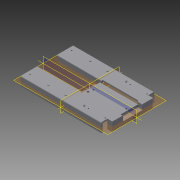
# Autodesk Inventor part: KarosserieDachTeil1
Saved by Autodesk Inventor 2015 (Build 190159000, 159)
## iProperties
Created: 2018-12-10
Part Number: KarosserieDachTeil1
Material: Generisch
Document SubType Name: Modeling
Designer: Boris
Density: 1 g/cm^3
Appearance: Vorgabe
Author: Boris
Autodesk Inventor part; units mm, degrees
sketch "Skizze1" plane through (0, 0, 0) normal (0, 0, 1) x (1, 0, 0)
  line L0 (-123.688, 77) -> (123.688, 77)
  line L1 (123.688, 77) -> (123.688, -77)
  line L2 (123.688, -77) -> (-123.688, -77)
  line L3 (-123.688, -77) -> (-123.688, 77)
  line L4 (-173.1632, 0) -> (173.1632, 0) projected
  line L5 (0, 107.8) -> (0, -107.8) projected
  point P0 (0, 0)
  dimension "d0" = 247.376
  dimension "d1" = 154
  constraints: 8 end point, 2 parallel, 1 horizontal, 1 perpendicular, 2 other
  measures "d0" distance of L1.end L2.end
  measures "d1" distance of L0.end L1.end
extrude "Extrusion1" add sketch "Skizze1" along normal mid plane 27
sketch "Skizze2" plane through (0, 0, -13.5) normal (0, 0, -1) x (-1, 0, 0)
  line L0 (123.688, -73) -> (-123.688, -73)
  line L1 (173.1632, 0) -> (-173.1632, 0) projected
  line L2 (123.688, -31) -> (-123.688, -31)
  line L3 (-123.688, -77) -> (123.688, -77) projected
  line L4 (123.688, 73) -> (-123.688, 73)
  line L5 (123.688, 31) -> (-123.688, 31)
  line L6 (123.688, -73) -> (123.688, -31)
  line L7 (0, -107.8) -> (0, 107.8) projected
  line L8 (-123.688, -73) -> (-123.688, -31)
  line L9 (123.688, 73) -> (123.688, 31)
  line L10 (-123.688, 73) -> (-123.688, 31)
  point P0 (0, 0)
  dimension "d4" = 4
  dimension "d5" = 42
  dimension "d8" = 123.688
  dimension "d13" = 123.688
  constraints: 16 end point, 4 symmetric about line, 1 horizontal, 1 parallel, 1 vertical
  measures "d4" distance between parallel lines of L3 L0
  measures "d5" distance between parallel lines of L0 L2
  measures "d8" distance between parallel lines of L7 L6
  measures "d13" distance between parallel lines of L8 L7
extrude "Extrusion2" cut sketch "Skizze2" against normal blind 23
sketch "Skizze3" plane through (0, 0, 13.5) normal (0, 0, 1) x (1, 0, 0)
  line L0 (-123.688, 31) -> (123.688, 31) projected
  line L1 (123.688, -31) -> (-123.688, -31) projected
  line L2 (-123.688, 28) -> (123.688, 28)
  line L3 (123.688, -28) -> (-123.688, -28)
  line L4 (-123.688, 28) -> (-123.688, -28)
  line L5 (-123.688, 77) -> (-123.688, -77) projected
  line L6 (123.688, 28) -> (123.688, -28)
  line L7 (123.688, -77) -> (123.688, 77) projected
  point P0 (0, 0)
  dimension "d11" = 3
  dimension "d12" = 3
  dimension "d14" = 247.376
  dimension "d15" = 247.376
  constraints: 8 end point, 2 collinear, 2 parallel
  measures "d11" distance between parallel lines of L0 L2
  measures "d12" distance between parallel lines of L1 L3
  measures "d14" distance between parallel lines of L4 L6
  measures "d15" distance between parallel lines of L7 L4
extrude "Extrusion3" cut sketch "Skizze3" against normal blind 23 contours L2 L6 L3 L4
sketch "Skizze4" plane through (-123.688, -73, -13.5) normal (0, 1, 0) x (1, 0, 0)
  line L0 (0, -23) -> (247.376, -23) projected
  line L1 (0, 0) -> (247.376, 0) projected
  line L2 (48.688, -23) -> (198.688, -23)
  line L3 (198.688, -23) -> (198.688, 0)
  line L4 (198.688, 0) -> (48.688, 0)
  line L5 (48.688, 0) -> (48.688, -23)
  line L6 (123.688, 5.4) -> (123.688, -32.4) projected
  point P0 (123.688, -13.5)
  dimension "d18" = 150
  constraints: 8 end point, 2 parallel, 2 point on line, 1 horizontal, 1 perpendicular, 1 other
  measures "d18" distance of L3.end L4.end
extrude "Extrusion4" cut sketch "Skizze4" against normal blind 2
sketch "Skizze5" plane through (-123.688, -31, -13.5) normal (0, -1, 0) x (1, 0, 0)
  line L0 (198.688, 0) -> (198.688, 23) projected
  line L1 (48.688, 23) -> (48.688, 0) projected
  line L2 (198.688, 0) -> (48.688, 0)
  line L3 (48.688, 0) -> (48.688, 23)
  line L4 (48.688, 23) -> (198.688, 23)
  line L5 (198.688, 23) -> (198.688, 0)
  point P0 (123.688, 13.5)
  constraints: 8 end point, 2 parallel, 1 horizontal, 1 perpendicular
extrude "Extrusion5" cut sketch "Skizze5" against normal blind 1
sketch "Skizze6" plane through (0, 0, 9.5) normal (0, 0, -1) x (-1, 0, 0)
  line L0 (75, -30) -> (-75, -30)
  line L1 (-75, -30) -> (-75, -75)
  line L2 (-75, -75) -> (75, -75)
  line L3 (75, -75) -> (75, -30)
  point P0 (0, 0)
  point P1 (-75, -30)
  point P2 (75, -75)
  constraints: 8 end point, 2 parallel, 1 horizontal, 1 perpendicular
extrude "Extrusion6" cut sketch "Skizze6" against normal blind 2
sketch "Skizze7" plane through (0, 0, -9.5) normal (0, 0, 1) x (1, 0, 0)
  line L0 (-123.688, 28) -> (123.688, 28) projected
  line L1 (-123.688, -28) -> (-123.688, 28) projected
  line L2 (123.688, -28) -> (-123.688, -28) projected
  line L3 (123.688, 28) -> (123.688, -28) projected
  line L4 (123.688, -28) -> (-123.688, -28) projected
  line L5 (123.688, 28) -> (-123.688, 28)
  line L6 (-123.688, 28) -> (-123.688, -28)
  line L7 (-123.688, -28) -> (123.688, -28)
  line L8 (123.688, -28) -> (123.688, 28)
  line L9 (123.688, 31) -> (123.688, -31) projected
  point P0 (0, 0)
  constraints: 8 end point, 2 parallel, 1 horizontal
extrude "Extrusion7" add sketch "Skizze7" along normal blind 8
sketch "Skizze10" plane through (0, 0, 13.5) normal (0, 0, 1) x (1, 0, 0)
  line L0 (-173.1632, 0) -> (173.1632, 0) projected
  circle A0 centre (104.872, 60.5) radius 1.5
  circle A1 centre (56.117, 60.5) radius 1.5
  line L1 (123.688, 28) -> (123.688, 77) projected
  line L2 (123.688, 77) -> (-123.688, 77) projected
  circle A2 centre (-113.279, 60.5) radius 1.5
  circle A3 centre (104.872, -60.5) radius 1.5
  circle A4 centre (56.117, -60.5) radius 1.5
  circle A5 centre (-113.279, -60.5) radius 1.5
  point P0 (0, 0)
  dimension "d36" = 3
  dimension "d37" = 3
  dimension "d38" = 18.816
  dimension "d39" = 16.5
  dimension "d40" = 48.755
  dimension "d41" = 16.5
  dimension "d42" = 3
  dimension "d44" = 169.396
  dimension "d45" = 16.5
  constraints: 6 centre point, 3 symmetric about line, 3 other
  measures "d36" diameter of A0
  measures "d37" diameter of A1
  measures "d38" distance from line of L1 A0.centre
  measures "d39" distance from line of L2 A0.centre
  measures "d40" distance of A1.centre A0.centre
  measures "d41" distance from line of L2 A1.centre
  measures "d42" diameter of A2
  measures "d44" distance of A1.centre A2.centre
  measures "d45" distance from line of L2 A2.centre
extrude "Extrusion10" cut sketch "Skizze10" against normal blind 13
sketch "Skizze12" plane through (-123.688, 28, 13.5) normal (0, -1, 0) x (1, 0, 0)
  line L0 (0, -15) -> (247.376, -15) projected
  line L1 (247.376, -15) -> (0, -15) projected
  line L2 (0, -15) -> (247.376, -15) projected
  line L3 (123.688, -15) -> (0, -15)
  line L4 (0, -15) -> (0, -48.1421)
  line L5 (123.688, -15) -> (0, -48.1421)
  point P0 (123.688, -13.5)
  dimension "d49" = 15
  constraints: 6 end point, 1 collinear, 1 midpoint, 1 vertical
  measures "d49" angle of L5 L0
extrude "Extrusion11" cut sketch "Skizze12" along normal up to surface (56 mm away)
sketch "Skizze16" plane through (0, 0, -13.5) normal (0, 0, -1) x (-1, 0, 0)
  line L0 (44.7846, 28) -> (123.688, 28) projected
  line L1 (123.688, 28) -> (123.688, 31) projected
  line L2 (123.688, 31) -> (-123.688, 31) projected
  line L3 (-123.688, 31) -> (-123.688, -31) projected
  line L4 (-123.688, -31) -> (-75, -31) projected
  line L5 (-75, -31) -> (-75, -30) projected
  line L6 (-75, -30) -> (75, -30) projected
  line L7 (75, -30) -> (75, -31) projected
  line L8 (75, -31) -> (123.688, -31) projected
  line L9 (123.688, -31) -> (123.688, -28) projected
  line L10 (123.688, -28) -> (44.7846, -28) projected
  line L11 (44.7846, -28) -> (44.7846, 28) projected
  point P0 (0, 0)
extrude "Extrusion14" cut sketch "Skizze16" against normal blind 8
sketch "Skizze17" plane through (0, -28, -1.5) normal (-0.258819, 0, 0.9659258) x (0.9659258, 0, 0.258819)
  circle A0 centre (-6, 10) radius 1.5
  line L0 (-171.7663, 28) -> (172.5427, 28) projected
  line L1 (0, 0) -> (-15.4548, 0) projected
  line L2 (0, 56) -> (0, 0) projected
  circle A1 centre (-6, 46) radius 1.5
  point P0 (0.3882, 28)
  dimension "d64" = 3
  dimension "d66" = 10
  dimension "d67" = 6
  constraints: 2 centre point, 1 symmetric about line, 1 other
  measures "d64" diameter of A0
  measures "d66" distance from line of L1 A0.centre
  measures "d67" distance from line of L2 A0.centre
extrude "Extrusion15" cut sketch "Skizze17" against normal blind 8
sketch "Skizze18" plane through (-123.688, 77, 13.5) normal (0, 1, 0) x (1, 0, 0)
  line L0 (247.376, 27) -> (0, 27) projected
  line L1 (247.376, 0) -> (233.376, 0)
  line L2 (233.376, 0) -> (233.376, 27)
  line L3 (233.376, 27) -> (247.376, 27)
  line L4 (247.376, 27) -> (247.376, 0)
  point P0 (123.688, 13.5)
  dimension "d70" = 14
  constraints: 8 end point, 2 parallel, 1 horizontal, 1 perpendicular, 1 point on line
  measures "d70" distance of L2.end L3.end
extrude "Extrusion16" cut sketch "Skizze18" against normal blind 18
mirror "Spiegeln1" about plane through (0, 0, 0) normal (0, 1, 0) of "Extrusion16"
sketch "Skizze19" plane through (0, 0, 13.5) normal (0, 0, 1) x (1, 0, 0)
  line L0 (123.688, 28) -> (123.688, 59) projected
  line L1 (123.688, 59) -> (109.688, 59) projected
  line L2 (108.872, 55) -> (119.688, 55)
  line L3 (119.688, 55) -> (119.688, 28)
  line L4 (123.188, 28) -> (123.188, 58.5)
  line L5 (123.188, 58.5) -> (108.872, 58.5)
  line L6 (123.188, 28) -> (119.688, 28)
  line L7 (-123.688, 28) -> (123.688, 28) projected
  line L8 (108.872, 55) -> (108.872, 58.5)
  point P0 (0, 0)
  dimension "d73" = 4
  dimension "d74" = 0.5
  constraints: 12 end point, 1 collinear, 1 vertical
  measures "d73" distance between parallel lines of L1 L2
  measures "d74" distance between parallel lines of L0 L4
extrude "Extrusion17" add sketch "Skizze19" against normal up to surface (27 mm away)
mirror "Spiegeln2" about plane through (0, 0, 0) normal (0, 1, 0) of "Extrusion17"
sketch "Skizze20" plane through (0, 0, -5.5) normal (0, 0, -1) x (-1, 0, 0)
  line L0 (-123.188, -28) -> (-119.688, -28) projected
  line L1 (-119.688, 28) -> (-123.188, 28) projected
  line L2 (-123.188, -28) -> (-123.188, 28)
  line L3 (0, 28) -> (-123.688, 28) projected
  line L4 (-119.688, 28) -> (-119.688, -28)
  point P0 (0, 0)
  constraints: 4 end point, 2 perpendicular
extrude "Extrusion18" add sketch "Skizze20" along normal up to surface (8 mm away)
sketch "Skizze21" plane through (0, 0, 13.5) normal (0, 0, 1) x (1, 0, 0)
  circle A0 centre (44.117, 60.5) radius 2.5
  circle A1 centre (56.117, 60.5) radius 1.5 projected
  line L0 (109.688, 77) -> (-123.688, 77) projected
  point P0 (0, 0)
  dimension "d80" = 5
  dimension "d81" = 8
  constraints: 1 centre point
  measures "d80" diameter of A0
extrude "Extrusion19" add sketch "Skizze21" along normal blind 2.5 contours A0
sketch "Skizze22" plane through (44.117, 60.5, 16) normal (0, 0, 1) x (1, 0, 0)
  line L0 (2.9126, -0.7189) -> (-2.9126, -0.7189)
  line L1 (-2.8965, 0.7811) -> (2.8965, 0.7811)
  arc A0 (2.9126, -0.7189) -> (2.8965, 0.7811) centre (0, 0) ccw
  arc A1 (-2.8965, 0.7811) -> (-2.9126, -0.7189) centre (0, 0) ccw
  point P0 (-44.117, -60.5)
  constraints: 4 end point, 4 point on circle, 2 centre point, 1 coincident, 1 horizontal, 1 parallel
extrude "Extrusion20" cut sketch "Skizze22" against normal blind 1
mirror "Spiegeln3" about plane through (0, 0, 0) normal (0, 1, 0) of "Extrusion19", "Extrusion20"
thread "Gewinde1" size "M3x0.5" class "6H" standard "ANSI Metric M Profile" full length
thread "Gewinde2" size "M3x0.5" class "6H" standard "ANSI Metric M Profile" full length
thread "Gewinde3" size "M3x0.5" class "6H" standard "ANSI Metric M Profile" full length
thread "Gewinde4" size "M3x0.5" class "6H" standard "ANSI Metric M Profile" full length
thread "Gewinde5" size "M3x0.5" class "6H" standard "ANSI Metric M Profile" full length
thread "Gewinde6" size "M3x0.5" class "6H" standard "ANSI Metric M Profile" full length
sketch "Skizze24" plane through (0, 0, -1.5) normal (0, 0, 1) x (1, 0, 0)
  line L0 (-173.1632, 0) -> (173.1632, 0) projected
  line L1 (0, -107.8) -> (0, 107.8) projected
  line L2 (123.688, -28) -> (0, -28) projected
  line L3 (0, 28) -> (115, 28)
  line L4 (115, 28) -> (115, -28)
  line L5 (115, -28) -> (0, -28)
  line L6 (0, -28) -> (0, 28)
  circle A0 centre (105, 0) radius 1.8
  circle A1 centre (10, 0) radius 1.8
  point P0 (0, 0)
  dimension "d99" = 115
  dimension "d101" = 3.6
  dimension "d102" = 3.6
  constraints: 8 end point, 2 centre point, 2 parallel, 1 horizontal, 1 perpendicular, 1 point on line
  measures "d99" distance of L4.end L5.end
  measures "d101" diameter of A0
  measures "d102" diameter of A1
extrude "Extrusion21" cut sketch "Skizze24" against normal blind 10 contours A1 L0 | L0 A1 | A0 L0 | L0 A0
thread "Gewinde7" size "M4x0.7" class "6H" standard "ANSI Metric M Profile" full length
thread "Gewinde8" size "M4x0.7" class "6H" standard "ANSI Metric M Profile" full length
sketch "Skizze25" plane through (0, 0, 13.5) normal (0, 0, 1) x (1, 0, 0)
  circle A0 centre (56.117, 60.5) radius 1.5 projected
  circle A1 centre (-113.279, 60.5) radius 1.5 projected
  line L0 (0, 107.8) -> (0, -107.8) projected
  line L1 (109.688, 77) -> (-123.688, 77) projected
  line L2 (-7.5, 60.5) -> (-8.75, 58.3349)
  line L3 (-8.75, 58.3349) -> (-11.25, 58.3349)
  line L4 (-11.25, 58.3349) -> (-12.5, 60.5)
  line L5 (-12.5, 60.5) -> (-11.25, 62.6651)
  line L6 (-11.25, 62.6651) -> (-8.75, 62.6651)
  line L7 (-8.75, 62.6651) -> (-7.5, 60.5)
  line L8 (-57.5, 60.5) -> (-58.75, 58.3349)
  line L9 (-58.75, 58.3349) -> (-61.25, 58.3349)
  line L10 (-61.25, 58.3349) -> (-62.5, 60.5)
  line L11 (-62.5, 60.5) -> (-61.25, 62.6651)
  line L12 (-61.25, 62.6651) -> (-58.75, 62.6651)
  line L13 (-58.75, 62.6651) -> (-57.5, 60.5)
  point P0 (0, 0)
  point P1 (-10, 60.5)
  point P2 (-60, 60.5)
  constraints: 24 end point, 26 other
extrude "Extrusion22" add sketch "Skizze25" along normal blind 1.5 contours L2 L3 L4 L5 L6 L7 | L8 L9 L10 L11 L12 L13
mirror "Spiegeln4" about plane through (0, 0, 0) normal (0, 1, 0) of "Extrusion22"
fillet "Rundung1" radius 3 2 edges at (-7, 77, 13.5) (-7, -77, 13.5)
fillet "Rundung2" radius 2 2 edges at (0, -28, 13.5) (0, 28, 13.5)
fillet "Rundung3" radius 2 2 edges at (61.844, -28, -1.5) (61.844, 28, -1.5)
fillet "Rundung4" radius 2 4 edges at (3.7321, -28, -0.5) (-7.4641, -28, -3.5) (3.7321, 28, -0.5) (-7.4641, 28, -3.5)
sketch "Skizze26" plane through (0, 0, -5.5) normal (0, 0, -1) x (-1, 0, 0)
  circle A0 centre (-10, 0) radius 1.8 projected
  line L0 (-10, 0) -> (-10, -12.5)
  circle A1 centre (-7, -12.5) radius 3
  point P0 (0, 0)
  dimension "d121" = 12.5
  dimension "d123" = 6
  constraints: 2 end point, 1 centre point, 1 tangent, 1 vertical
  measures "d121" distance of L0.start L0.end
  measures "d123" diameter of A1
extrude "Extrusion23" cut sketch "Skizze26" against normal blind 7 contours A1
sketch "Skizze27" plane through (0, 0, 13.5) normal (0, 0, 1) x (1, 0, 0)
  line L0 (106.9687, 31.5) -> (8.4073, 31.5)
  line L1 (8.4073, -31.5) -> (106.9687, -31.5)
  line L2 (-173.1632, 0) -> (173.1632, 0) projected
  line L3 (123.688, -26) -> (123.688, 26) projected
  arc A0 (109.8468, -29.3465) -> (109.8468, 29.3465) centre (10.0732, 0) ccw
  line L4 (-123.688, 31) -> (119.688, 31) projected
  line L5 (57.688, 31) -> (57.688, -31.5)
  arc A1 (5.5292, 29.3465) -> (5.5292, -29.3465) centre (105.3028, 0) ccw
  arc A2 (109.8468, 29.3465) -> (106.9687, 31.5) centre (106.9687, 28.5) ccw
  arc A3 (106.9687, -31.5) -> (109.8468, -29.3465) centre (106.9687, -28.5) ccw
  arc A4 (5.5292, -29.3465) -> (8.4073, -31.5) centre (8.4073, -28.5) ccw
  arc A5 (8.4073, 31.5) -> (5.5292, 29.3465) centre (8.4073, 28.5) ccw
  point P0 (0, 0)
  point P1 (109.188, 31.5)
  point P2 (6.188, -31.5)
  point P3 (6.188, 31.5)
  point P4 (109.188, -31.5)
  dimension "d126" = 63
  dimension "d128" = 103
  dimension "d129" = 104
  dimension "d130" = 3
  constraints: 16 point on circle, 8 tangent, 6 centre point, 6 end point, 5 point on line, 3 equal radius, 1 horizontal, 1 midpoint, 1 parallel, 1 symmetric about line, 2 other
  measures "d126" distance of point (109.188, -31.5) point (109.188, 31.5)
  measures "d128" distance of point (6.188, -31.5) point (109.188, -31.5)
  measures "d129" radius of A0
  measures "d130" radius of A2
extrude "Extrusion24" cut sketch "Skizze27" against normal up to surface (15 mm away)
sketch "Skizze28" plane through (0, 0, -1.5) normal (0, 0, 1) x (1, 0, 0)
  line L0 (110.7707, 26) -> (110.7707, -26)
  line L1 (110.233, 28) -> (110.7707, 26)
  line L2 (110.7707, -26) -> (110.233, -28)
  line L3 (110.233, 28) -> (0, 28)
  line L4 (110.233, -28) -> (5.143, -28)
  line L5 (0, 26) -> (0, -26)
  line L6 (0, 28) -> (0, 26)
  circle A0 centre (10, 0) radius 1.8 projected
  circle A1 centre (7, -12.5) radius 3 projected
  circle A2 centre (105, 0) radius 1.8 projected
  line L7 (5.143, -28) -> (0, -28)
  line L8 (0, -26) -> (0, -28)
  point P0 (0, 0)
  point P1 (4.6053, 26)
  point P2 (4.6053, -26)
  point P3 (5.143, 28)
  constraints: 18 end point, 3 vertical, 2 horizontal
extrude "Extrusion25" add sketch "Skizze28" along normal blind 8
sketch "Skizze29" plane through (0, 0, -5.5) normal (0, 0, -1) x (-1, 0, 0)
  line L0 (-110.7707, 26) -> (-110.7707, -26) projected
  line L1 (0, 26) -> (0, -26) projected
  line L2 (-107.7707, 26) -> (-107.7707, -26)
  line L3 (-3, 26) -> (-3, -26)
  line L4 (-107.7707, -26) -> (-3, -26)
  line L5 (-5.143, -28) -> (-110.233, -28) projected
  line L6 (-3, 26) -> (-107.7707, 26)
  point P0 (0, 0)
  dimension "d136" = 3
  dimension "d137" = 3
  constraints: 8 end point, 4 parallel
  measures "d136" distance between parallel lines of L0 L2
  measures "d137" distance between parallel lines of L1 L3
extrude "Extrusion26" cut sketch "Skizze29" against normal blind 9
sketch "Skizze30" plane through (0, 0, 6.5) normal (0, 0, 1) x (1, 0, 0)
  line L0 (110.233, 28) -> (110.7707, 28)
  line L1 (110.7707, 28) -> (110.7707, 26)
  line L2 (110.233, 28) -> (110.7707, 26)
  line L3 (110.233, -28) -> (110.7707, -28)
  line L4 (110.7707, -28) -> (110.7707, -26)
  line L5 (110.233, -28) -> (110.7707, -26)
  point P0 (0, 0)
  constraints: 12 end point, 1 horizontal, 1 perpendicular
extrude "Extrusion27" add sketch "Skizze30" against normal up to surface (8 mm away)
fillet "Rundung7" radius 3 5 edges at (110.7707, -27.4142, -0.9142) (110.7707, -28, 3.5) (110.7707, 27.4142, -0.9142) (110.7707, 28, 3.5) (110.7707, 0, -1.5)
sketch "Skizze31" plane through (0, 0, -1.5) normal (0, 0, 1) x (1, 0, 0)
  line L0 (5.143, 28) -> (110.233, 28) projected
  arc A0 (110.233, 28) -> (109.8468, 29.3465) centre (10.0732, 0) ccw projected
  arc A1 (109.8468, 29.3465) -> (108.627, 31) centre (106.9687, 28.5) ccw projected
  line L1 (6.749, 31) -> (108.627, 31) projected
  arc A2 (6.749, 31) -> (5.5292, 29.3465) centre (8.4073, 28.5) ccw projected
  arc A3 (5.5292, 29.3465) -> (5.143, 28) centre (105.3028, 0) ccw projected
  line L2 (110.233, -28) -> (5.143, -28) projected
  arc A4 (5.143, -28) -> (5.5292, -29.3465) centre (105.3028, 0) ccw projected
  arc A5 (5.5292, -29.3465) -> (5.8092, -30) centre (8.4073, -28.5) ccw projected
  line L3 (75, -30) -> (5.8092, -30) projected
  line L4 (75, -31) -> (75, -30) projected
  line L5 (108.627, -31) -> (75, -31) projected
  arc A6 (108.627, -31) -> (109.8468, -29.3465) centre (106.9687, -28.5) ccw projected
  arc A7 (109.8468, -29.3465) -> (110.233, -28) centre (10.0732, 0) ccw projected
  line L6 (5.143, 28) -> (110.233, 28) projected
  arc A8 (109.8468, 29.3465) -> (108.627, 31) centre (106.9687, 28.5) ccw projected
  line L7 (6.749, 31) -> (108.627, 31) projected
  arc A9 (6.749, 31) -> (5.5292, 29.3465) centre (8.4073, 28.5) ccw projected
  arc A10 (5.5292, 29.3465) -> (5.143, 28) centre (105.3028, 0) ccw projected
  line L8 (110.233, -28) -> (5.143, -28) projected
  arc A11 (5.143, -28) -> (5.5292, -29.3465) centre (105.3028, 0) ccw projected
  arc A12 (5.5292, -29.3465) -> (5.8092, -30) centre (8.4073, -28.5) ccw projected
  line L9 (75, -30) -> (5.8092, -30) projected
  line L10 (75, -31) -> (75, -30) projected
  line L11 (108.627, -31) -> (75, -31) projected
  arc A13 (108.627, -31) -> (109.8468, -29.3465) centre (106.9687, -28.5) ccw projected
  arc A14 (109.8468, -29.3465) -> (110.233, -28) centre (10.0732, 0) ccw projected
  arc A15 (110.233, 28) -> (109.8468, 29.3465) centre (10.0732, 0) ccw projected
  point P0 (0, 0)
extrude "Extrusion28" cut sketch "Skizze31" against normal up to surface (4 mm away)
sketch "Skizze32" plane through (0, 0, -5.5) normal (0, 0, -1) x (-1, 0, 0)
  line L0 (-5.143, 28) -> (-110.233, 28)
  line L1 (-110.233, 28) -> (-110.233, -28)
  line L2 (-110.233, -28) -> (-5.143, -28)
  line L3 (-5.143, -28) -> (-5.143, 28)
  point P0 (0, 0)
  dimension "d11" = 3
  dimension "d12" = 3
  dimension "d14" = 247.376
  dimension "d15" = 247.376
  constraints: 8 end point, 2 parallel, 1 horizontal, 1 perpendicular
extrude "Extrusion29" cut sketch "Skizze32" against normal up to surface (9 mm away)
fillet "Rundung8" radius 2 3 edges at (-58.4695, 31, -5.5) (-99.344, -31, -5.5) (-75, -30.5, -5.5)
fillet "Rundung9" radius 2 2 edges at (4.0715, -26, -5.5) (4.0715, 26, -5.5)
fillet "Rundung10" radius 1 4 edges at (2.5715, 28, 6.5) (2.5715, -28, 6.5) (112.0019, -28, 6.5) (112.0019, 28, 6.5)
fillet "Rundung11" radius 1 3 edges at (0, -27.7071, 6.7929) (0, 27.7071, 6.7929) (0, 0, 6.5)
sketch "Skizze33" plane through (0, 0, -5.5) normal (0, 0, -1) x (-1, 0, 0)
  line L0 (-119.688, -31) -> (-108.627, -31) projected
  line L1 (123.688, 31) -> (-6.749, 31) projected
  line L2 (-110.233, -31) -> (-3.0118, -31)
  line L3 (-3.0118, -31) -> (-3.0118, 31)
  line L4 (-3.0118, 31) -> (-110.233, 31)
  line L5 (-110.233, 31) -> (-110.233, -31)
  point P0 (0, 0)
  constraints: 8 end point, 2 parallel, 2 point on line, 1 horizontal, 1 perpendicular
extrude "Extrusion30" cut sketch "Skizze33" against normal up to surface (9 mm away)
chamfer "Fase3" distance 7 distance2 6 1 edges at (3, 0, -5.5) measured on face at (3, 0, -5)
fillet "Rundung12" radius 4 1 edges at (-3, 0, -5.5)
fillet "Rundung13" radius 3 1 edges at (110.233, 0, -5.5)
fillet "Rundung14" radius 1 4 edges at (6.749, 31, 6.5) (108.627, 31, 6.5) (5.8092, -30, 7.5) (108.627, -31, 6.5)
